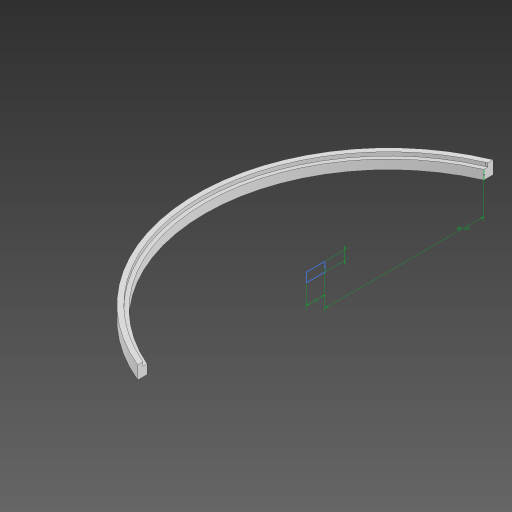
# Autodesk Inventor part: Деталь2
Saved by Autodesk Inventor 2023 (Build 270158000, 158)
## iProperties
Created: 2025-08-05
Part Number: Деталь2
Material: Типовые
Document SubType Name: Modeling
Designer: daa
Density: 1 g/cm^3
Appearance: По умолчанию
Author: daa
Autodesk Inventor part; units mm, degrees
ref_plane "YZ Plane" through (0, 0, 0) normal (1, 0, 0) x (0, 1, 0)
ref_plane "XZ Plane" through (0, 0, 0) normal (0, 1, 0) x (-1, 0, 0)
ref_plane "XY Plane" through (0, 0, 0) normal (0, 0, 1) x (1, 0, 0)
sketch "Эскиз1" plane through (0, 0, 0) normal (0, 1, 0) x (-1, 0, 0)
  line L0 (0, 0) -> (0, -192.264)
  arc A0 (0, -192.264) -> (0, 0) centre (-39.6817, -96.132) ccw
  line L1 (0, 0) -> (0, -5)
  line L2 (0, -192.264) -> (0, -187.264)
  arc A1 (0, -187.264) -> (0, -5) centre (-39.6817, -96.132) ccw
  dimension "d0" = 192.264
  dimension "d1" = 104
  dimension "d2" = 5
  dimension "d3" = 5
  dimension "d4" = 99.3966
  constraints: 6 end point, 4 point on circle, 2 centre point, 2 point on line, 1 vertical
  measures "d0" distance of L0.start L0.end
  measures "d1" radius of A0
  measures "d2" distance of L0.start L1.end
  measures "d3" distance of L0.end L2.end
  measures "d4" radius of A1
extrude "Выдавливание1" add sketch "Эскиз1" along normal blind 7 contours A0 L0 A1
sketch "Эскиз2" plane through (0, 7, 0) normal (0, 1, 0) x (1, 0, 0)
  arc A0 (0, 187.264) -> (0, 5) centre (39.6817, 96.132) ccw projected
  arc A1 (-0.7985, 189.0977) -> (-0.7985, 3.1663) centre (39.6817, 96.132) ccw
  line L0 (-0.7985, 3.1663) -> (0, 2.8227)
  line L1 (-0.7985, 189.0977) -> (0, 189.4413)
  line L2 (0, 0) -> (0, 5) projected
  line L3 (0, 2.8227) -> (0, 5)
  line L4 (0, 189.4413) -> (0, 187.264)
  arc A2 (0, 187.264) -> (0, 5) centre (39.6817, 96.132) ccw
  dimension "d8" = 2
  constraints: 8 end point, 4 point on circle, 2 centre point, 1 collinear, 1 concentric, 1 vertical
  measures "d8" radial gap between concentric circles of A0 A1
extrude "Выдавливание2" cut sketch "Эскиз2" against normal blind 2
sketch "Эскиз3" plane through (0, 0, 0) normal (1, 0, 0) x (0, 1, 0)
  line L0 (5, -91.132) -> (0, -91.132)
  line L1 (0, -91.132) -> (0, -101.132)
  line L2 (0, -101.132) -> (5, -101.132)
  line L3 (5, -101.132) -> (5, -91.132)
  line L4 (0, -187.264) -> (5, -187.264) projected
  point P0 (2.5, -187.264)
  point P1 (2.5, -101.132)
  dimension "d11" = 5
  dimension "d12" = 10
  dimension "d13" = 86.132
  constraints: 8 end point, 2 midpoint, 2 parallel, 1 horizontal, 1 perpendicular
  measures "d11" distance of L2.end L1.end
  measures "d12" distance of L1.end L0.end
  measures "d13" distance of point (2.5, -187.264) point (2.5, -101.132)
